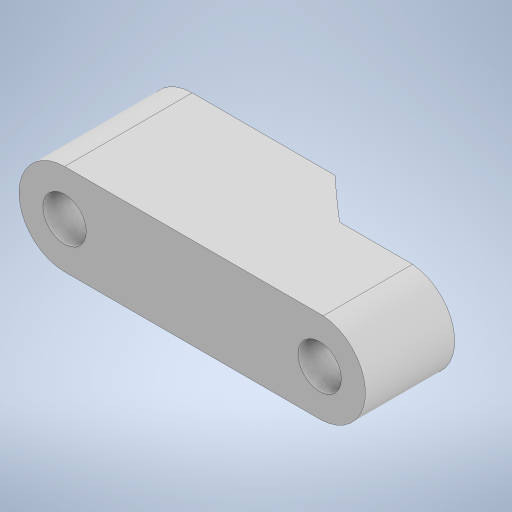
# Autodesk Inventor part: ArmMuscle
Saved by Autodesk Inventor 2023 (Build 270158000, 158)
## iProperties
Created: 2023-06-03
Part Number: ArmMuscle
Material: Ogólny
Document SubType Name: Modeling
Designer: Kamil
Density: 1 g/cm^3
Appearance: Domyślna
Author: Kamil
Autodesk Inventor part; units mm, degrees
ref_plane "YZ Plane" through (0, 0, 0) normal (1, 0, 0) x (0, 1, 0)
ref_plane "XZ Plane" through (0, 0, 0) normal (0, 1, 0) x (-1, 0, 0)
ref_plane "XY Plane" through (0, 0, 0) normal (0, 0, 1) x (1, 0, 0)
sketch "Szkic1" plane through (0, 0, 0) normal (0, 0, 1) x (1, 0, 0)
  line L0 (21.6558, 4.5742) -> (1.0948, 4.5742)
  circle A0 centre (1.3753, 0.9987) radius 3.5755
  circle A1 centre (1.3753, 0.9994) radius 1.7002
  line L1 (1.0948, -2.5758) -> (21.6558, -2.5758)
  circle A2 centre (21.3721, 1.0041) radius 3.5808
  circle A3 centre (21.3763, 0.9967) radius 1.6973
  point P0 (0, 0)
  point P1 (-2.1997, -2.5758)
  point P2 (1.3753, 4.5742)
  point P3 (1.2909, -2.5758)
  point P4 (21.4558, -2.5758)
  point P5 (21.6483, 4.5742)
  constraints: 4 centre point, 4 end point
extrude "Wyciągnięcie proste1" add sketch "Szkic1" along normal blind 10 contours A2 L0 | A2 L1 A0 L0 | A0 picked at (21.9206, 3.8831)
sketch "Szkic2" plane through (0, 0, 0) normal (0, 0, -1) x (-1, 0, 0)
  arc A0 (-17.3627, -1.0651) -> (-17.8563, 4.5702) centre (-20.4272, 1.5058) ccw projected
  line L0 (-17.3627, -1.0651) -> (-21.219, -5.6617) projected
  circle A1 centre (-21.3763, 0.9967) radius 1.6973 projected
  line L1 (-21.3763, 0.9967) -> (-16.4424, 1.8548)
  line L2 (-16.4424, 1.8548) -> (-14.9646, 2.1118)
  circle A2 centre (-21.3763, 0.9967) radius 6.508
  arc A3 (-1.2909, -2.5758) -> (-1.3753, 4.5742) centre (-1.3753, 0.9987) ccw projected
  line L3 (-21.6483, 4.5742) -> (-1.3753, 4.5742) projected
  arc A4 (-21.6483, 4.5742) -> (-21.4558, -2.5758) centre (-21.3721, 1.0041) ccw projected
  line L4 (-1.2909, -2.5758) -> (-21.4558, -2.5758) projected
  circle A5 centre (-1.3753, 0.9994) radius 1.7002 projected
  circle A6 centre (-21.3763, 0.9967) radius 1.6973 projected
  point P0 (0, 0)
  point P1 (-15.9366, -2.5758)
  point P2 (-15.9399, 4.5742)
  dimension "d2" = 1.5
  constraints: 4 end point, 1 coincident, 1 point on circle, 3 other
  measures "d2" distance of L1.end L2.end
extrude "Wyciągnięcie proste2" cut sketch "Szkic2" against normal blind 3 contours L0 L4 A4 L3 A2 L2 A0 | A0 L2 A2 L4 L0
chamfer "Faza1" distance 3 angle 45 1 edges at (14.8684, 0.9997, 0)
